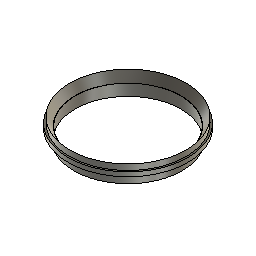
closure (Autodesk Fusion 360 design; units mm, degrees)
Autodesk Fusion 360 part; units mm, degrees
sketch "Skizze14" plane through (0, 0, 0) normal (0, 0, 1) x (1, 0, 0)
  circle A0 centre (0, 0) radius 38.2
  circle A1 centre (0, 0) radius 37.2
  dimension "d43" = 76.4
  dimension "d44" = -1
  constraint coincident A0.centre A1.centre
  measures "d43" diameter of A0
extrude "Extrusion11" add sketch "Skizze14" against normal blind 10 makes body 1
sketch "Skizze15" plane through (0, 0, 0) normal (0, 1, 0) x (1, 0, 0)
sketch "Skizze16" plane through (0, 0, 0) normal (0, 0, 1) x (1, 0, 0)
  circle A0 centre (0, 0) radius 42.1
  circle A1 centre (0, 0) radius 38.2
  dimension "d47" = 84.2
  dimension "d48" = -3.9
  constraint coincident A0.centre A1.centre
  measures "d47" diameter of A0
extrude "Extrusion12" add sketch "Skizze16" against normal blind 3 bodies 1
sketch "Skizze1" plane through (0, 0, 0) normal (0, 0, 1) x (1, 0, 0)
  circle A0 centre (0, 0) radius 42.1
  circle A1 centre (0, 0) radius 40.9
  dimension "d1" = 84.2
  dimension "d2" = -1.2
  constraint coincident A0.centre A1.centre
  measures "d1" diameter of A0
sketch "Skizze17" plane through (0, 0, 0) normal (0, 1, 0) x (1, 0, 0)
sketch "Skizze18" plane through (0, 0, 0) normal (0, 0, 1) x (1, 0, 0)
  circle A0 centre (0, 0) radius 40.9
  dimension "d53" = 81.8
  constraint coincident A0.centre origin
  measures "d53" diameter of A0
extrude "Extrusion13" cut sketch "Skizze18" against normal blind 1.8 bodies 1
sketch "Skizze19" plane through (0, 0, 0) normal (0, 0, 1) x (1, 0, 0)
ref_plane "Arbeitsebene2" through (0, 0, -1.8) normal (0, 0, 1) x (1, 0, 0)
sketch "Skizze20" plane through (0, 0, -1.8) normal (0, 0, 1) x (1, 0, 0)
sketch "Skizze21" plane through (0, 0, 0) normal (0, 1, 0) x (1, 0, 0)
ref_plane "Arbeitsebene4" through (0, 0, -1.8) normal (0, 0, 1) x (1, 0, 0)
sketch "Skizze26" plane through (0, 0, -1.8) normal (0, 0, 1) x (1, 0, 0)
sketch "Skizze27" plane through (0, 0, 0) normal (0, 1, 0) x (1, 0, 0)
sketch "Skizze28" plane through (0, 0, 0) normal (0, 1, 0) x (1, 0, 0)
sketch "Skizze29" plane through (0, 0, 0) normal (0, 1, 0) x (1, 0, 0)
  line L0 (42, 0) -> (41.7559, 0)
  line L1 (40.8986, 1.8065) -> (40.8986, -3.9935)
  line L2 (40.8986, 1.8065) -> (37, 1.8065)
  line L3 (40.8986, -3.9935) -> (37, 1.8065)
  dimension "d67" = 5.8
  constraint horizontal L0
  constraint perpendicular L1 L2
  measures "d67" distance of L1.start L1.end
revolve "Drehen3" add sketch "Skizze29" angle 360 about axis through (0, 0, 1.75) along (0, 0, 1) separate body makes body 2
sketch "Skizze30" plane through (0, 0, 0) normal (0, 0, 1) x (1, 0, 0)
sketch "Skizze22" plane through (0, 0, 0) normal (0, 1, 0) x (1, 0, 0)
sketch "Skizze23" plane through (0, 0, -1.8) normal (0, 0, 1) x (1, 0, 0)
ref_plane "Arbeitsebene3" through (0, -1.8, 0) normal (0, 1, 0) x (0, 0, 1)
equation "d44 = 1 mm - 2 mm"
